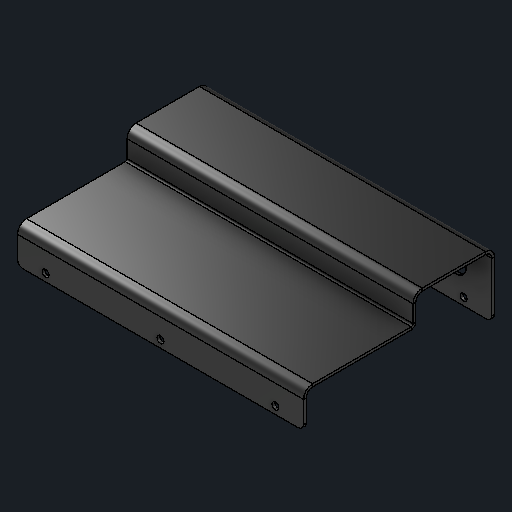
# Autodesk Inventor part: Top Shell
Saved by Autodesk Inventor 2026.2 (Build 302298000, 298)
## iProperties
Created: 2026-06-19
Part Number: Top Shell
Material: Steel, Carbon
Document SubType Name: Sheet Metal
Designer: JoshuaEah
Density: 7.85 g/cm^3
Sheet Metal Rule: Default_mm
Appearance: Glossy - Black
Author: JoshuaEah
Autodesk Inventor part; units mm, degrees
ref_plane "YZ Plane" through (0, 0, 0) normal (1, 0, 0) x (0, 1, 0)
ref_plane "XZ Plane" through (0, 0, 0) normal (0, 1, 0) x (-1, 0, 0)
sketch "Sketch1" plane through (0, 0, 0) normal (0, 1, 0) x (-1, 0, 0)
  line L0 (0, 0) -> (-158, 0)
  line L1 (-158, 0) -> (-158, -62)
  line L2 (-158, -62) -> (0, -62)
  line L3 (0, -62) -> (0, 0)
  dimension "d0" = 62
  dimension "d1" = 158
  measures "d0" distance of L0.end L1.end
  measures "d1" distance of L1.end L2.end
extrude "Plate1" add sketch "Sketch1" along normal blind 1.5
sketch "Sketch2" plane through (0, 0, -60.5) normal (0, 0, -1) x (-1, 0, 0)
  line L0 (-158, 0) -> (0, 0)
  line L1 (0, 0) -> (0, 17)
  line L2 (0, 17) -> (-158, 17)
  line L3 (-158, 17) -> (-158, 0)
  constraints: 6 end point, 1 horizontal, 1 perpendicular, 1 vertical
edge flange "Flange1" height 17 angle 90 thickness 1.5 bend radius 1 thickness toward (0, 0, -1) relief tear relief width 1.5 relief depth 0.75 edges at (79, 1.5, -62) wall of the first edge with corners at (158, 0, -60.5) (0, 0, -60.5) (0, 17, -60.5) (158, 17, -60.5)
bend "Bend1"
corner "Corner1"
sketch "Sketch3" plane through (0, 1.5, -1.5) normal (0, 0, 1) x (1, 0, 0)
  line L0 (158, 0) -> (0, 0)
  line L1 (0, 0) -> (0, -20)
  line L2 (0, -20) -> (158, -20)
  line L3 (158, -20) -> (158, 0)
  constraints: 6 end point, 1 horizontal, 1 perpendicular, 1 vertical
edge flange "Flange2" height 20 angle 90 thickness 1.5 bend radius 3.5 thickness toward (0, 0, 1) relief tear relief width 1.5 relief depth 0.75 edges at (79, 0, 0) wall of the first edge with corners at (158, 1.5, -1.5) (0, 1.5, -1.5) (0, -18.5, -1.5) (158, -18.5, -1.5)
bend "Bend2"
corner "Corner2"
sketch "Sketch4" plane through (158, 15.5, -60.5) normal (0, 1, 0) x (-1, 0, 0)
  line L0 (158, 0) -> (0, 0)
  line L1 (0, 0) -> (0, -45)
  line L2 (0, -45) -> (158, -45)
  line L3 (158, -45) -> (158, 0)
  constraints: 6 end point, 1 horizontal, 1 perpendicular, 1 vertical
edge flange "Flange3" height 45 angle 90 thickness 1.5 bend radius 3.5 thickness toward (0, 1, 0) relief tear relief width 1.5 relief depth 0.75 edges at (79, 17, -62) wall of the first edge with corners at (0, 15.5, -60.5) (158, 15.5, -60.5) (158, 15.5, -105.5) (0, 15.5, -105.5)
bend "Bend3"
corner "Corner3"
sketch "Sketch5" plane through (158, 17, -104) normal (0, 0, -1) x (-1, 0, 0)
  line L0 (158, 0) -> (0, 0)
  line L1 (0, 0) -> (0, -35.5)
  line L2 (0, -35.5) -> (158, -35.5)
  line L3 (158, -35.5) -> (158, 0)
  constraints: 6 end point, 1 horizontal, 1 perpendicular, 1 vertical
edge flange "Flange4" height 35.5 angle 90 thickness 1.5 bend radius 3.5 thickness toward (0, 0, -1) relief tear relief width 1.5 relief depth 0.75 edges at (79, 15.5, -105.5) wall of the first edge with corners at (0, 17, -104) (158, 17, -104) (158, -18.5, -104) (0, -18.5, -104)
bend "Bend4"
corner "Corner4"
sketch "Hole Patterns" plane through (158, -18.5, -105.5) normal (0, 0, -1) x (-1, 0, 0)
  line L0 (158, 30.5) -> (0, 30.5) construction
  line L1 (0, 0) -> (0, 30.5) construction
  line L2 (158, 0) -> (0, 0) construction
  line L3 (158, 30.5) -> (158, 0) construction
  line L4 (79, 30.5) -> (79, 0)
  circle A0 centre (79, 4.125) radius 2.875
  circle A1 centre (19.675, 18.675) radius 7.825
  circle A2 centre (135.5, 17) radius 5
  dimension "d54" = 5.75
  dimension "d55" = 4.125
  dimension "d57" = 15.65
  dimension "d58" = 19.675
  dimension "d59" = 18.675
  dimension "d77" = 10
  dimension "d78" = 17
  dimension "d79" = 22.5
  constraints: 3 centre point, 2 end point, 2 midpoint, 1 point on line
  measures "d54" diameter of A0
  measures "d55" distance from line of L2 A0.centre
  measures "d57" diameter of A1
  measures "d58" distance from line of L1 A1.centre
  measures "d59" distance from line of L2 A1.centre
  measures "d77" diameter of A2
  measures "d78" distance from line of L2 A2.centre
  measures "d79" distance from line of L3 A2.centre
ref_plane "Work Plane1" through (158, -18.5, -52.75) normal (0, 0, -1) x (-1, 0, 0)
hole "Mounting Hole (Rear)" at (79, -14.375, -105.5) direction (0, 0, 1) diameter 3.81 depth 1.5 clearance for "Oval Head Machine Screw" size "#6" standard "Ansi Unified Screw Threads"
pattern_linear "Mounting Holes (Rear)" count 3 spacing 63.475 along (1, 0, 0) of "Mounting Hole (Rear)" first direction both ways yes
mirror "Mounting Holes (Front)" about plane through (158, -18.5, -52.75) normal (0, 0, -1) of "Mounting Hole (Rear)", "Mounting Holes (Rear)"
hole "1/4\" Jack Mounting Hole" at (138.325, 0.175, -105.5) direction (0, 0, 1) diameter 11 depth 1.5
pattern_linear "1/4\" Jack Mounts" count 4 spacing 21.55 along (-1, 0, 0) of "1/4\" Jack Mounting Hole"
hole "DC Input Jack" at (22.5, -1.5, -105.5) direction (0, 0, 1) diameter 10 depth 1.5
pattern_linear "DC Input Jacks" count 2 spacing 35 along (1, 0, 0) of "DC Input Jack"
fillet "Fillet1" radius 3 4 edges at (158, -18.5, -0.75) (0, -18.5, -0.75) (0, -18.5, -104.75) (158, -18.5, -104.75)
equation "\"d2\" = Thickness"
equation "\"d3\" = BendReliefWidth"
equation "\"d4\" = BendReliefDepth"
equation "\"d5\" = MinimumRemnant"
equation "\"d6\" = TransitionRadius"
equation "\"d10\" = CornerReliefSize"
equation "\"d11\" = GapSize"
equation "\"d12\" = JacobiRadiusSize"
equation "\"d13\" = BendReliefWidth"
equation "\"d14\" = BendReliefDepth"
equation "\"d15\" = MinimumRemnant"
equation "\"d16\" = TransitionRadius"
equation "\"d20\" = CornerReliefSize"
equation "\"d21\" = GapSize"
equation "\"d22\" = JacobiRadiusSize"
equation "\"d23\" = BendReliefWidth"
equation "\"d24\" = BendReliefDepth"
equation "\"d25\" = MinimumRemnant"
equation "\"d26\" = TransitionRadius"
equation "\"d30\" = CornerReliefSize"
equation "\"d31\" = GapSize"
equation "\"d32\" = JacobiRadiusSize"
equation "\"d33\" = BendReliefWidth"
equation "\"d34\" = BendReliefDepth"
equation "\"d35\" = MinimumRemnant"
equation "\"d36\" = TransitionRadius"
equation "\"d40\" = CornerReliefSize"
equation "\"d41\" = GapSize"
equation "\"d42\" = JacobiRadiusSize"
equation "\"BendRadius\" = Thickness"
equation "\"BendReliefWidth\" = Thickness"
equation "\"BendReliefDepth\" = 0.5 * Thickness"
equation "\"CornerReliefSize\" = 4 * Thickness"
equation "\"MinimumRemnant\" = 2 * Thickness"
equation "\"TransitionRadius\" = BendRadius"
equation "\"JacobiRadiusSize\" = BendRadius"
equation "\"GapSize\" = Thickness"
equation "\"Thickness\" = 1.5"
body "Solid1"
